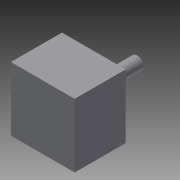
# Autodesk Inventor part: dop_krepl_k_sponke_ne_motora
Saved by Autodesk Inventor 2015 (Build 190159000, 159)
## iProperties
Created: 2016-05-14
Part Number: dop_krepl_k_sponke_ne_motora
Material: Generic
Document SubType Name: Modeling
Designer: Andreas
Density: 1 g/cm^3
Appearance: Default
Author: Andreas
Autodesk Inventor part; units mm, degrees
ref_plane "YZ Plane" through (0, 0, 0) normal (1, 0, 0) x (0, 1, 0)
ref_plane "XZ Plane" through (0, 0, 0) normal (0, 1, 0) x (-1, 0, 0)
ref_plane "XY Plane" through (0, 0, 0) normal (0, 0, 1) x (1, 0, 0)
sketch "Sketch1" plane through (0, 0, 0) normal (0, 1, 0) x (-1, 0, 0)
  line L0 (0, 0) -> (0, -25)
  line L1 (0, -25) -> (25, -25)
  line L2 (25, -25) -> (25, 0)
  line L3 (25, 0) -> (0, 0)
  point P0 (0, -12.5)
  point P1 (12.5, 0)
  dimension "d0" = 25
  dimension "d1" = 25
  constraints: 8 end point, 2 midpoint, 2 perpendicular, 1 horizontal, 1 vertical
  measures "d0" distance of L0.start L0.end
  measures "d1" distance of L0.end L1.end
extrude "Extrusion2" add sketch "Sketch1" along normal blind 20
sketch "Sketch2" plane through (0, 20, 0) normal (0, 1, 0) x (1, 0, 0)
  circle A0 centre (-12.5, 12.5) radius 2.5
  line L0 (0, 0) -> (0, 25) projected
  line L1 (-25, 0) -> (0, 0) projected
  dimension "d7" = 5
  dimension "d18" = 12.5
  dimension "d19" = 12.5
  constraints: 1 centre point
  measures "d7" diameter of A0
  measures "d18" distance from line of L0 A0.centre
  measures "d19" distance from line of L1 A0.centre
extrude "Extrusion3" add sketch "Sketch2" along normal blind 17
sketch "Sketch3" plane through (0, 20, 0) normal (0, 1, 0) x (1, 0, 0)
  circle A0 centre (-12.5, 12.5) radius 3.5
  line L0 (0, 0) -> (0, 25) projected
  line L1 (-25, 0) -> (0, 0) projected
  dimension "d10" = 7
  dimension "d20" = 12.5
  dimension "d21" = 12.5
  constraints: 1 centre point
  measures "d10" diameter of A0
  measures "d20" distance from line of L0 A0.centre
  measures "d21" distance from line of L1 A0.centre
extrude "Extrusion4" add sketch "Sketch3" along normal blind 2.75
sketch "Sketch4" plane through (-12.5, 37, -12.5) normal (0, 1, 0) x (1, 0, 0)
  circle A0 centre (0, 0) radius 1
  point P0 (12.5, -12.5)
  dimension "d13" = 2
  constraints: 1 centre point
  measures "d13" diameter of A0
extrude "Extrusion5" cut sketch "Sketch4" against normal blind 4
thread "Thread1" size "M2x0.4" class "6H" standard "ANSI Metric M Profile" full length
body "Solid2"
